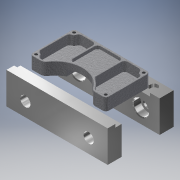
# Autodesk Inventor part: CAM Mania Tutorial
Saved by Autodesk Inventor 2017 (Build 210142000, 142)
## iProperties
Created: 2013-03-01
Part Number: CAM Mania Tutorial
Material: Generic
Document SubType Name: Modeling
Designer: Autodesk, Inc.
Density: 1 g/cm^3
Appearance: Aluminum - Polished
Author: Autodesk, Inc.
Autodesk Inventor part; units mm, degrees
ref_plane "YZ Plane" through (0, 0, 0) normal (1, 0, 0) x (0, 1, 0)
ref_plane "XZ Plane" through (0, 0, 0) normal (0, 1, 0) x (-1, 0, 0)
ref_plane "XY Plane" through (0, 0, 0) normal (0, 0, 1) x (1, 0, 0)
sketch "Sketch1" plane through (0, 0, 0) normal (0, 0, 1) x (1, 0, 0)
  line L0 (-16.1606, 0) -> (92.3606, 0) projected
  line L1 (0, -24.2615) -> (0, 56.6691) projected
  line L2 (10.3555, 0) -> (3.175, 0)
  arc A0 (76.2, 41.275) -> (73.025, 44.45) centre (73.025, 41.275) ccw
  line L3 (3.175, 44.45) -> (73.025, 44.45)
  arc A1 (3.175, 44.45) -> (0, 41.275) centre (3.175, 41.275) ccw
  line L4 (0, 3.175) -> (0, 41.275)
  arc A2 (0, 3.175) -> (3.175, 0) centre (3.175, 3.175) ccw
  line L5 (73.025, 0) -> (65.8445, 0)
  arc A3 (73.025, 0) -> (76.2, 3.175) centre (73.025, 3.175) ccw
  line L6 (76.2, 41.275) -> (76.2, 3.175)
  arc A4 (60.6097, 2.7557) -> (15.5903, 2.7557) centre (38.1, -12.7) ccw
  arc A5 (60.6097, 2.7557) -> (65.8445, 0) centre (65.8445, 6.35) ccw
  arc A6 (10.3555, 0) -> (15.5903, 2.7557) centre (10.3555, 6.35) ccw
  line L7 (51.054, 44.196) -> (50.8, 44.45)
  line L8 (25.4, 44.45) -> (25.146, 44.196)
  point P0 (0, 0)
  point P1 (38.1, 44.45)
  dimension "d0" = 44.45
  dimension "d1" = 76.2
  dimension "d3" = 12.7
  dimension "d4" = 27.305
  dimension "d5" = 3.175
  dimension "d6" = 6.35
  constraints: 14 end point, 14 point on circle, 13 tangent, 7 centre point, 3 equal radius, 2 point on line, 2 vertical, 1 midpoint, 1 parallel, 1 vertical alignment
  measures "d0" distance of L3.start L2.end
  measures "d1" distance of L6.start L4.end
  measures "d3" vertical distance of A4.centre L2.end
  measures "d4" radius of A4
  measures "d5" radius of A3
  measures "d6" radius of A5
extrude "Extrusion1" add sketch "Sketch1" along normal blind 12.7 contours A2 L1 A1 L3 A0 L6 A3 L0 A5 A4 A6
sketch "Sketch2" plane through (0, 0, 0) normal (0, 0, -1) x (-1, 0, 0)
  line L0 (-76.2, 41.275) -> (-76.2, 3.175) projected
  line L1 (-50.8, 50.8739) -> (-25.4, 50.8739)
  line L2 (-25.4, 50.8739) -> (-25.4, 5.0654)
  line L3 (-25.4, 5.0654) -> (-50.8, 5.0654)
  line L4 (-50.8, 5.0654) -> (-50.8, 50.8739)
  line L5 (-38.1, 50.8739) -> (-38.1, 61.5092) construction
  line L6 (0, 41.275) -> (0, 3.175) projected
  point P0 (0, 0)
  dimension "d10" = 25.4
  dimension "d210" = 38.1
  constraints: 10 end point, 3 parallel, 1 horizontal, 1 midpoint, 1 perpendicular
  measures "d10" distance of L1.start L1.end
  measures "d210" distance between parallel lines of L6 L5
extrude "Extrusion2" cut sketch "Sketch2" against normal blind 6.35
sketch "Sketch3" plane through (0, 0, 12.7) normal (0, 0, 1) x (1, 0, 0)
  arc A0 (23.7998, 39.2183) -> (20.3708, 42.6473) centre (20.3708, 39.2183) ccw
  arc A1 (22.251, 11.4727) -> (23.7998, 14.3403) centre (20.3708, 14.3403) ccw
  arc A2 (55.8292, 42.6386) -> (52.4002, 39.2096) centre (55.8292, 39.2096) ccw
  arc A3 (4.0664, 38.01) -> (1.6002, 34.7189) centre (5.0292, 34.7189) ccw
  arc A4 (9.5178, 42.6473) -> (6.2244, 40.1732) centre (9.5178, 39.2183) ccw
  arc A5 (1.6002, 9.5134) -> (4.0664, 6.2223) centre (5.0292, 9.5134) ccw
  arc A6 (6.2223, 4.0664) -> (9.5134, 1.6002) centre (9.5134, 5.0292) ccw
  arc A7 (72.1336, 6.1526) -> (74.5998, 9.4437) centre (71.1708, 9.4437) ccw
  arc A8 (66.7074, 1.6002) -> (69.9877, 4.0303) centre (66.7074, 5.0292) ccw
  arc A9 (74.5998, 34.7189) -> (72.1336, 38.01) centre (71.1708, 34.7189) ccw
  arc A10 (69.9768, 40.169) -> (66.6847, 42.6386) centre (66.6847, 39.2096) ccw
  arc A11 (69.9768, 40.169) -> (72.1336, 38.01) centre (73.025, 41.0573) ccw
  arc A12 (72.1336, 6.1526) -> (69.9877, 4.0303) centre (73.025, 3.1053) ccw
  line L0 (9.5134, 1.6002) -> (10.3555, 1.6002)
  arc A13 (6.2223, 4.0664) -> (4.0664, 6.2223) centre (3.175, 3.175) ccw
  line L1 (1.6002, 34.7189) -> (1.6002, 9.5134)
  arc A14 (4.0664, 38.01) -> (6.2244, 40.1732) centre (3.175, 41.0573) ccw
  line L2 (20.3708, 42.6473) -> (9.5178, 42.6473)
  line L3 (23.7998, 14.3403) -> (23.7998, 39.2183)
  arc A15 (22.251, 11.4727) -> (14.2712, 3.6614) centre (38.1, -12.7) ccw
  arc A16 (10.3555, 1.6002) -> (14.2712, 3.6614) centre (10.3555, 6.35) ccw
  arc A17 (28.829, 42.543) -> (25.4, 39.114) centre (28.829, 39.114) ccw
  arc A18 (25.4, 18.2766) -> (29.8122, 14.9916) centre (28.829, 18.2766) ccw
  line L4 (66.6847, 42.6386) -> (55.8292, 42.6386)
  line L5 (74.5998, 9.4437) -> (74.5998, 34.7189)
  arc A19 (46.3878, 14.9916) -> (50.8, 18.2766) centre (47.371, 18.2766) ccw
  arc A20 (50.8, 39.114) -> (47.371, 42.543) centre (47.371, 39.114) ccw
  line L6 (65.8425, 1.6002) -> (66.7074, 1.6002)
  line L7 (47.371, 42.543) -> (28.829, 42.543)
  line L8 (25.4, 39.114) -> (25.4, 18.2766)
  line L9 (50.8, 18.2766) -> (50.8, 39.114)
  line L10 (76.2, 3.175) -> (76.2, 41.275) projected
  line L11 (65.8445, 0) -> (73.025, 0) projected
  line L12 (73.025, 44.45) -> (3.175, 44.45) projected
  line L13 (0, 41.275) -> (0, 3.175) projected
  arc A21 (60.6097, 2.7557) -> (15.5903, 2.7557) centre (38.1, -12.7) ccw projected
  arc A22 (60.6097, 2.7557) -> (65.8445, 0) centre (65.8445, 6.35) ccw projected
  arc A23 (10.3555, 0) -> (15.5903, 2.7557) centre (10.3555, 6.35) ccw projected
  arc A24 (0, 3.175) -> (3.175, 0) centre (3.175, 3.175) ccw projected
  line L14 (10.3555, 0) -> (3.175, 0)
  arc A25 (73.025, 0) -> (76.2, 3.175) centre (73.025, 3.175) ccw projected
  line L15 (52.4002, 39.2096) -> (52.4002, 14.3403)
  line L16 (38.1, 42.543) -> (38.1, 52.1949) construction
  arc A26 (52.4002, 14.3403) -> (53.949, 11.4727) centre (55.8292, 14.3403) ccw
  arc A27 (61.9929, 3.5678) -> (65.8425, 1.6002) centre (65.8425, 6.35) ccw
  arc A28 (61.9929, 3.5678) -> (53.949, 11.4727) centre (38.1, -12.7) ccw
  arc A29 (46.3878, 14.9916) -> (29.8122, 14.9916) centre (38.1, -12.7) ccw
  point P0 (0, 0)
  point P1 (0, 0)
  point P2 (52.4002, 12.42)
  point P3 (59.9268, 1.6002)
  point P4 (59.1703, 1.6002)
  dimension "d13" = 1.6002
  dimension "d14" = 1.6002
  dimension "d166" = 1.6002
  dimension "d168" = 1.6002
  dimension "d169" = 3.175
  dimension "d170" = 3.175
  dimension "d171" = 3.175
  dimension "d172" = 3.1053
  dimension "d173" = 3.3927
  dimension "d174" = 3.3927
  dimension "d175" = 3.175
  dimension "d176" = 1.6002
  dimension "d179" = 1.6002
  dimension "d180" = 1.8027
  dimension "d181" = 1.907
  dimension "d182" = 1.8114
  dimension "d183" = 3.175
  dimension "d184" = 25.4
  dimension "d190" = 3.429
  dimension "d191" = 3.175
  dimension "d192" = 3.429
  dimension "d193" = 3.429
  dimension "d194" = 3.429
  dimension "d195" = 3.429
  dimension "d196" = 3.429
  dimension "d197" = 3.429
  dimension "d198" = 3.175
  dimension "d199" = 3.429
  dimension "d201" = 3.429
  dimension "d204" = 1.6002
  dimension "d205" = 38.1
  dimension "d206" = 3.429
  dimension "d207" = 3.429
  dimension "d208" = 3.429
  dimension "d209" = 3.429
  constraints: 50 point on circle, 34 tangent, 26 end point, 25 centre point, 7 parallel, 4 equal radius, 3 concentric, 3 point on line, 1 collinear, 1 midpoint, 1 perpendicular
  measures "d13" horizontal distance of point (0, 0) L1.end
  measures "d14" vertical distance of L0.start point (0, 0)
  measures "d166" distance between parallel lines of L8 L3
  measures "d168" distance between parallel lines of L10 L5
  measures "d169" radius of A11
  measures "d170" distance from line of L10 A11.centre
  measures "d171" distance from line of L10 A12.centre
  measures "d172" distance from line of L11 A12.centre
  measures "d173" distance from line of L12 A11.centre
  measures "d174" distance from line of L12 A14.centre
  measures "d175" distance from line of L13 A14.centre
  measures "d176" radial gap between concentric circles of A21 A15
  measures "d179" distance between parallel lines of L13 L1
  measures "d180" distance between parallel lines of L12 L2
  measures "d181" distance between parallel lines of L12 L7
  measures "d182" distance between parallel lines of L12 L4
  measures "d183" radius of A13
  measures "d184" distance between parallel lines of L9 L8
  measures "d190" radius of A3
  measures "d191" radius of A14
  measures "d192" radius of A4
  measures "d193" radius of A5
  measures "d194" radius of A6
  measures "d195" radius of A10
  measures "d196" radius of A9
  measures "d197" radius of A7
  measures "d198" radius of A12
  measures "d199" radius of A8
  measures "d201" radius of A1
  measures "d204" distance between parallel lines of L15 L9
  measures "d205" distance between parallel lines of L13 L16
  measures "d206" radius of A17
  measures "d207" radius of A20
  measures "d208" radius of A19
  measures "d209" radius of A18
extrude "Extrusion3" cut sketch "Sketch3" against normal blind 9.525 contours L3 A1 A15 A16 L0 A6 A13 A5 L1 A3 A14 A4 L2 A0 | L4 A10 A11 A9 L5 A7 A12 A8 L6 A27 A28 A26 L15 A2
extrude "Extrusion4" cut sketch "Sketch3" against normal blind 3.175
chamfer "Chamfer2" distance 0.254 angle 45 28 edges at (0, 22.225, 12.7) (0.9299, 0.9299, 12.7) (6.7653, 0, 12.7) (13.3134, 0.731, 12.7) (38.1, 14.605, 12.7) (62.8866, 0.731, 12.7) (69.4347, 0, 12.7) (75.2701, 0.9299, 12.7) (76.2, 22.225, 12.7) (75.2701, 43.5201, 12.7) (38.1, 44.45, 12.7) (0.9299, 43.5201, 12.7) (0, 22.225, 0) (0.9299, 43.5201, 0) (14.2875, 44.45, 0) (0.9299, 0.9299, 0) (6.7653, 0, 0) (13.3134, 0.731, 0) (19.9638, 7.7118, 0) (56.2362, 7.7118, 0) (62.8866, 0.731, 0) (69.4347, 0, 0) (75.2701, 0.9299, 0) (76.2, 22.225, 0) (75.2701, 43.5201, 0) (61.9125, 44.45, 0) (25.4, 27.9609, 0) (50.8, 27.9609, 0)
hole "Hole1" at (3.175, 3.175, 12.7) direction (0, 0, -1) diameter 2.6416 depth 6.35 thread size "6-32 UNC" class "2B" standard "ANSI Unified Screw Threads"
hole "Hole2" at (3.175, 3.175, 6.35) direction (0, 0, -1) diameter 2.7178 depth 2.3813 tip angle 118
chamfer "Chamfer3" distance 0.254 angle 45 1 edges at (3.175, 4.4958, 12.7)
pattern_linear "Rectangular Pattern1" count 2 spacing 69.85 along (1, 0, 0) count 2 spacing 38.1 along (0, 1, 0) of "Hole1", "Hole2", "Chamfer3"
chamfer "Chamfer1" distance 0.254 angle 45 33 edges at (2.2852, 36.7752, 12.7) (5.4228, 38.8149, 12.7) (7.4582, 41.9599, 12.7) (14.9443, 42.6473, 12.7) (22.7955, 41.643, 12.7) (23.7998, 26.7793, 12.7) (23.3878, 12.7107, 12.7) (17.8803, 7.9561, 12.7) (12.568, 2.147, 12.7) (9.9344, 1.6002, 12.7) (7.4571, 2.2852, 12.7) (5.4201, 5.4201, 12.7) (2.2852, 7.4571, 12.7) (1.6002, 22.1161, 12.7) (26.4043, 41.5386, 12.7) (38.1, 42.543, 12.7) (49.7957, 41.5386, 12.7) (50.8, 28.6953, 12.7) (49.4188, 15.5262, 12.7) (58.3602, 7.9163, 12.7) (26.7812, 15.5262, 12.7) (25.4, 28.6953, 12.7) (61.257, 42.6386, 12.7) (68.7425, 41.9526, 12.7) (70.7788, 38.8134, 12.7) (73.9148, 36.7752, 12.7) (74.5998, 22.0813, 12.7) (53.4045, 41.6343, 12.7) (52.4002, 26.7749, 12.7) (66.275, 1.6002, 12.7) (68.7486, 2.2739, 12.7) (70.7923, 5.3627, 12.7) (73.9148, 7.3874, 12.7)
ref_plane "Work Plane1" through (0, 0, 13.97) normal (0, 0, 1) x (1, 0, 0)
sketch "Sketch4" plane through (0, 0, 13.97) normal (0, 0, 1) x (1, 0, 0)
  line L0 (-3.175, -3.175) -> (79.375, -3.175)
  line L1 (79.375, -3.175) -> (79.375, 47.625)
  line L2 (79.375, 47.625) -> (-3.175, 47.625)
  line L3 (-3.175, 47.625) -> (-3.175, -3.175)
  line L4 (3.175, 0) -> (10.3555, 0) projected
  line L5 (0, 41.275) -> (0, 3.175) projected
  point P0 (0, 0)
  dimension "d62" = 82.55
  dimension "d63" = 50.8
  dimension "d64" = 3.175
  dimension "d65" = 3.175
  constraints: 8 end point, 2 parallel, 1 horizontal, 1 perpendicular
  measures "d62" distance of L0.start L0.end
  measures "d63" distance of L2.end L0.start
  measures "d64" distance from line of L5 L0.start
  measures "d65" distance from line of L0.start L4
extrude "Extrusion5" add sketch "Sketch4" against normal blind 19.05 separate body
ref_plane "Work Plane2" through (88.9, -3.175, 13.97) normal (1, 0, 0) x (0, 0, -1)
sketch "Sketch5" plane through (88.9, -3.175, 13.97) normal (1, 0, 0) x (0, 0, -1)
  line L0 (19.05, 50.8) -> (19.05, 0) projected
  line L1 (0, 50.8) -> (19.05, 50.8) projected
  line L2 (15.875, 58.42) -> (47.625, 58.42)
  line L3 (47.625, 58.42) -> (47.625, 44.45)
  line L4 (47.625, 44.45) -> (15.875, 44.45)
  line L5 (15.875, 44.45) -> (15.875, 58.42)
  line L6 (15.875, -7.62) -> (47.625, -7.62)
  line L7 (47.625, -7.62) -> (47.625, 6.35)
  line L8 (47.625, 6.35) -> (19.05, 6.35)
  line L9 (15.875, 0) -> (15.875, -7.62)
  line L10 (0, 0) -> (19.05, 0) projected
  line L11 (15.875, 0) -> (19.05, 0)
  line L12 (19.05, 0) -> (19.05, 6.35)
  point P0 (13.97, 3.175)
  dimension "d69" = 13.97
  dimension "d70" = 31.75
  dimension "d71" = 3.175
  dimension "d72" = 6.35
  dimension "d96" = 31.75
  dimension "d97" = 13.97
  constraints: 20 end point, 4 parallel, 3 perpendicular, 2 horizontal, 2 point on line
  measures "d69" distance of L2.end L3.end
  measures "d70" distance of L2.start L2.end
  measures "d71" distance from line of L4.end L0
  measures "d72" distance from line of L1 L4.end
  measures "d96" distance of L6.start L6.end
  measures "d97" distance of L6.end L7.end
extrude "Extrusion6" add sketch "Sketch5" against normal blind 101.6 separate body contours L1 L5 L2 L3 L4 L0 | L0 L4 L5 L1
sketch "Sketch6" plane through (88.9, 41.275, -1.905) normal (0, 0, 1) x (1, 0, 0)
  arc A0 (-84.963, 7.62) -> (-92.075, 7.62) centre (-88.519, 7.62) ccw
  line L0 (-84.963, 7.62) -> (-84.963, 6.35)
  line L1 (-84.963, 6.35) -> (-16.637, 6.35)
  line L2 (-16.637, 6.35) -> (-16.637, 7.62)
  arc A1 (-9.525, 7.62) -> (-16.637, 7.62) centre (-13.081, 7.62) ccw
  line L3 (-9.525, 7.62) -> (-9.525, 0)
  line L4 (-9.525, 0) -> (-92.075, 0)
  line L5 (-92.075, 0) -> (-92.075, 7.62)
  line L6 (-101.6, 0) -> (-101.6, 13.97) projected
  line L7 (0, 0) -> (-101.6, 0) projected
  point P0 (-88.9, -41.275)
  point P1 (-88.9, 0)
  dimension "d75" = 82.55
  dimension "d76" = 9.525
  dimension "d77" = 6.35
  dimension "d78" = 3.556
  dimension "d79" = 3.556
  dimension "d80" = 7.62
  constraints: 12 end point, 4 point on circle, 4 tangent, 3 perpendicular, 2 centre point, 2 parallel, 1 collinear, 1 horizontal, 1 horizontal alignment
  measures "d75" distance of L3.end L4.end
  measures "d76" distance between parallel lines of L5 L6
  measures "d77" distance between parallel lines of L1 L4
  measures "d78" radius of A0
  measures "d79" radius of A1
  measures "d80" vertical distance of A1.centre L3.end
extrude "Extrusion7" cut sketch "Sketch6" against normal blind 3.175 bodies 3
sketch "Sketch7" plane through (88.9, 41.275, -33.655) normal (0, -1, 0) x (1, 0, 0)
  line L0 (-101.6, 0) -> (-101.6, 31.75) projected
  line L1 (0, 0) -> (-101.6, 0) projected
  point P0 (-88.9, 33.655)
  point P1 (-82.55, 13.97)
  point P2 (-19.05, 13.97)
  dimension "d83" = 19.05
  dimension "d84" = 63.5
  dimension "d85" = 13.97
  constraints: 1 horizontal alignment
  measures "d83" distance from line of point (-82.55, 13.97) L0
  measures "d84" distance of point (-19.05, 13.97) point (-82.55, 13.97)
  measures "d85" distance from line of point (-82.55, 13.97) L1
hole "Hole4" at (6.35, 41.275, -19.685) at (69.85, 41.275, -19.685) direction (0, 1, 0) diameter 10.16 end through all counterbore diameter 15.24 counterbore depth 7.62 bodies 3
chamfer "Chamfer4" distance 0.7937 angle 45 2 edges at (6.35, 41.275, -12.065) (69.85, 41.275, -12.065)
extrude "Extrusion8" add sketch "Sketch5" against normal blind 101.6 separate body contours L8 L7 L6 L9 L10 L0
sketch "Sketch8" plane through (88.9, 3.175, -5.08) normal (0, 1, 0) x (1, 0, 0)
  line L0 (0, 28.575) -> (0, 0) projected
  point P0 (-88.9, -5.08)
  point P1 (-19.05, 14.605)
  point P2 (-82.55, 14.605)
  dimension "d102" = 19.05
  dimension "d103" = 63.5
  dimension "d104" = 13.97
  measures "d102" distance from line of point (-19.05, 14.605) L0
  measures "d103" distance of point (-82.55, 14.605) point (-19.05, 14.605)
  measures "d104" vertical distance of point (-19.05, 14.605) L0.start
hole "Hole5" at (69.85, 3.175, -19.685) at (6.35, 3.175, -19.685) direction (0, -1, 0) diameter 10.16 end through all counterbore diameter 15.24 counterbore depth 7.62 bodies 4
chamfer "Chamfer5" distance 0.7937 angle 45 2 edges at (69.85, 3.175, -27.305) (6.35, 3.175, -27.305)
sketch "Sketch9" plane through (88.9, 41.275, -5.08) normal (0, 0, 1) x (1, 0, 0)
  line L0 (-92.075, 0) -> (-92.075, 7.62) projected
  line L1 (-84.963, 6.35) -> (-16.637, 6.35) projected
  line L2 (-92.075, 6.35) -> (-9.525, 6.35)
  line L3 (-9.525, 6.35) -> (-9.525, -44.45)
  line L4 (-9.525, -44.45) -> (-92.075, -44.45)
  line L5 (-92.075, -44.45) -> (-92.075, 6.35)
  point P0 (-88.9, -41.275)
  dimension "d115" = 82.55
  dimension "d116" = 50.8
  constraints: 8 end point, 2 parallel, 1 horizontal, 1 perpendicular, 1 point on line
  measures "d115" distance of L2.start L2.end
  measures "d116" distance of L4.end L2.start
extrude "Extrusion9" add sketch "Sketch9" along normal blind 4.953 separate body
sketch "Sketch10" plane through (88.9, 41.275, -0.127) normal (0, 0, 1) x (1, 0, 0)
  line L0 (-12.7, -38.1) -> (-12.7, 0)
  line L1 (-15.875, 3.175) -> (-85.725, 3.175)
  line L2 (-88.9, 0) -> (-88.9, -38.1)
  line L3 (-92.075, -44.45) -> (-9.525, -44.45) projected
  line L4 (-71.4647, -26.67) -> (-29.9449, -26.67) construction
  arc A0 (-37.5587, -36.6385) -> (-63.8508, -36.6385) centre (-50.7048, -40.3225) ccw
  line L5 (-85.725, -41.275) -> (-69.9653, -41.275)
  line L6 (-31.4443, -41.275) -> (-15.875, -41.275)
  arc A1 (-85.725, 3.175) -> (-88.9, 0) centre (-85.725, 0) ccw
  arc A2 (-88.9, -38.1) -> (-85.725, -41.275) centre (-85.725, -38.1) ccw
  arc A3 (-15.875, -41.275) -> (-12.7, -38.1) centre (-15.875, -38.1) ccw
  arc A4 (-12.7, 0) -> (-15.875, 3.175) centre (-15.875, 0) ccw
  arc A5 (-69.9653, -41.275) -> (-63.8508, -36.6385) centre (-69.9653, -34.925) ccw
  arc A6 (-37.5587, -36.6385) -> (-31.4443, -41.275) centre (-31.4443, -34.925) ccw
  point P0 (-88.9, -41.275)
  point P1 (-88.9, -41.275)
  point P2 (-12.7, -41.275)
  point P3 (-88.9, 3.175)
  point P4 (-64.324, -41.275)
  point P5 (-37.0855, -41.275)
  dimension "d119" = 44.45
  dimension "d120" = 76.2
  dimension "d121" = 3.175
  dimension "d122" = 3.175
  dimension "d123" = 14.605
  dimension "d124" = 27.305
  dimension "d125" = 3.175
  dimension "d126" = 6.35
  constraints: 16 point on circle, 13 tangent, 12 end point, 8 point on line, 7 centre point, 4 equal radius, 4 parallel, 2 horizontal, 2 perpendicular
  measures "d119" distance of point (-88.9, 3.175) point (-88.9, -41.275)
  measures "d120" distance of point (-88.9, -41.275) point (-12.7, -41.275)
  measures "d121" distance from line of L3 point (-88.9, -41.275)
  measures "d122" horizontal distance of point (-88.9, -41.275) L3.start
  measures "d123" distance from line of L4 point (-88.9, -41.275)
  measures "d124" diameter of A0
  measures "d125" radius of A1
  measures "d126" radius of A5
extrude "Extrusion10" add sketch "Sketch10" along normal blind 12.827 bodies 5
